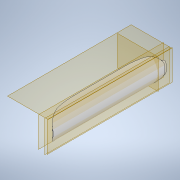
# Autodesk Inventor part: Deckel_Parachute_3
Saved by Autodesk Inventor 2020 (Build 240168000, 168)
## iProperties
Created: 2022-01-25
Part Number: Deckel_Parachute_3
Material: Generisch
Document SubType Name: Modeling
Designer: sp
Density: 1 g/cm^3
Appearance: Vorgabe
Author: sp
## iProperties of the stored document _3D-Druck.ipt
Created: 2022-05-02
Part Number: _3D-Druck
Material: Generisch
Document SubType Name: Modeling
Designer: sp
Density: 1 g/cm^3
Appearance: Vorgabe
Author: sp
Autodesk Inventor part; units mm, degrees
sketch "Skizze1" plane through (0, 0, 0) normal (0, 0, 1) x (1, 0, 0)
  circle A0 centre (0, 0) radius 31
  circle A1 centre (0, 0) radius 30
  dimension "d0" = 62
  dimension "d1" = 60
  constraints: 2 centre point, 2 coincident
  measures "d0" diameter of A0
  measures "d1" diameter of A1
extrude "Extrusion1" add sketch "Skizze1" along normal mid plane 300
sketch "Skizze2" plane through (0, 0, 0) normal (0, 1, 0) x (-1, 0, 0)
  line L0 (-11, 169.5773) -> (-11, -169.8146) construction
  line L1 (-74.8376, 0) -> (82.6362, 0) construction
  line L2 (-11, 75) -> (-11, -75)
  line L3 (-31, -150) -> (-31, 150) projected
  line L4 (31, 150) -> (-31, 150) projected
  line L5 (-31, -150) -> (31, -150) projected
  spline S0 degree 2 poles (-11, 75) (-17.8298, 136.4739) (-72.8449, 128.3193) knots 0 0 0 1 1 1
  spline S1 degree 2 poles (-11, -75) (-17.6171, -136.2673) (-74.8376, -130) knots 0 0 0 1 1 1
  line L6 (-72.8449, 128.3193) -> (-74.8376, -130)
  line L7 (-31, 120) -> (-31, 150)
  line L8 (-31, 150) -> (31, 150)
  line L9 (31, 150) -> (31, -150)
  line L10 (31, -150) -> (31, 150) projected
  line L11 (31, -150) -> (-31, -150)
  line L12 (-31, -150) -> (-31, -120)
  point P0 (0, 0)
  dimension "d4" = 11
  dimension "d5" = 150
  dimension "d6" = 30
  dimension "d7" = 30
  constraints: 18 end point, 5 point on line, 3 perpendicular, 2 collinear, 1 horizontal, 1 symmetric about line, 1 vertical, 6 other
  measures "d4" distance from line of point (0, 0) L0
  measures "d5" distance of L2.start L2.end
  measures "d6" distance from line of L7.start L4
  measures "d7" distance from line of L12.end L5
extrude "Extrusion3" cut sketch "Skizze2" along normal mid plane 100 contours S0 L3 L4 L9 L5 S1 L2
ref_plane "Arbeitsebene1" through (26.5, 0, 0) normal (1, 0, 0) x (0, 1, 0)
sketch "Skizze6" plane through (26.5, 0, 0) normal (1, 0, 0) x (0, 1, 0)
  line L0 (22.6784, 127.732) -> (-25.9609, 127.732)
  line L1 (-25.9609, 127.732) -> (-25.9609, 118.4744)
  line L2 (-25.9609, 118.4744) -> (22.6784, 118.4744)
  line L3 (22.6784, 118.4744) -> (22.6784, 127.732)
  point P0 (0, 0)
  dimension "d27" = 118.4744
  constraints: 8 end point, 2 parallel, 1 horizontal, 1 perpendicular
  measures "d27" distance from line of point (0, 0) L2
extrude "Extrusion5" cut sketch "Skizze6" against normal mid plane 10
ref_plane "Arbeitsebene3" through (0, 33.25, 0) normal (0, 1, 0) x (-1, 0, 0)
mirror "Spiegeln1" about plane through (0, 0, 0) normal (0, 0, 1) of "Extrusion5"
sketch "Skizze8" plane through (0, 33.25, 0) normal (0, 1, 0) x (-1, 0, 0)
  line L0 (-11, -75) -> (-11, 75) projected
  arc A0 (-11, 56.4646) -> (-14.2842, 92.4804) centre (-300.1138, 48.2584) ccw
  arc A1 (-11, 56.4646) -> (-14.2842, 92.4804) centre (-31.6354, 72.7405) ccw
  point P0 (0, 0)
  constraints: 4 point on circle, 2 centre point, 1 point on line
extrude "Extrusion6" cut sketch "Skizze8" against normal blind 65
mirror "Spiegeln2" about plane through (0, 0, 0) normal (0, 0, 1) of "Extrusion6"
ref_plane "Arbeitsebene4" through (0, 0, -103) normal (0, 0, 1) x (1, 0, 0)
sketch "Skizze9" plane through (0, 0, -103) normal (0, 0, 1) x (1, 0, 0)
  circle A0 centre (0, 0) radius 28
  circle A1 centre (0, 0) radius 30
  line L0 (0, 0) -> (55.2327, 31.8886)
  line L1 (0, 0) -> (53.5398, -30.9112)
  line L2 (0, -70.3595) -> (0, 85.9396) construction
  point P0 (24.2487, -14)
  point P1 (25.9808, -15)
  point P2 (25.9808, 15)
  point P3 (24.2487, 14)
  dimension "d36" = 56
  dimension "d37" = 60
  dimension "d38" = 60
  dimension "d39" = 60
  constraints: 6 end point, 2 centre point, 2 coincident, 1 point on line, 1 vertical
  measures "d36" diameter of A0
  measures "d37" diameter of A1
  measures "d38" angle of L0 L1
  measures "d39" angle of L0 L2
extrude "Extrusion7" add sketch "Skizze9" against normal blind 20 contours A0 L0 A1 L1 picked at (29.0396, 3.3572)
fillet "Rundung2" radius 5 2 edges at (25.1147, -14.5, -123) (25.1147, 14.5, -123)
ref_plane "Arbeitsebene5" through (30, 0, 0) normal (1, 0, 0) x (0, 1, 0)
sketch "Skizze10" plane through (30, 0, 0) normal (1, 0, 0) x (0, 1, 0)
  line L0 (0, 194.4728) -> (0, -210.0754) construction
  line L1 (-91.4107, 0) -> (91.4107, 0) construction
  line L2 (-4, 110) -> (4, 110)
  line L3 (4, 110) -> (4, 100)
  line L4 (4, 100) -> (-4, 100)
  line L5 (-4, 100) -> (-4, 110)
  point P0 (0, 0)
  point P1 (0, 0)
  dimension "d44" = 8
  dimension "d45" = 100
  dimension "d46" = 10
  constraints: 12 end point, 2 horizontal, 2 midpoint, 2 parallel, 2 point on line, 1 perpendicular, 1 vertical, 1 other
  measures "d44" distance of L3.end L4.end
  measures "d45" distance between parallel lines of L1 L4
  measures "d46" distance of L2.end L3.end
extrude "Extrusion8" add sketch "Skizze10" against normal blind 11
sketch "Skizze11" plane through (-30, -4, 100) normal (0, -1, 0) x (1, 0, 0)
  line L0 (51, 8) -> (57, 8)
  line L1 (57, 8) -> (57, 2)
  line L2 (57, 2) -> (51, 2)
  line L3 (51, 2) -> (51, 8)
  line L4 (59.7321, 10) -> (49, 10) projected
  line L5 (49, 0) -> (49, 10) projected
  point P0 (30, -100)
  point P1 (0, 10)
  dimension "d49" = 2
  dimension "d50" = 6
  dimension "d51" = 6
  dimension "d52" = 2
  constraints: 8 end point, 2 parallel, 1 horizontal, 1 perpendicular
  measures "d49" distance between parallel lines of L4 L0
  measures "d50" distance of L2.end L0.start
  measures "d51" distance of L0.start L0.end
  measures "d52" distance between parallel lines of L3 L5
extrude "Extrusion9" cut sketch "Skizze11" against normal blind 12
ref_plane "Arbeitsebene6" through (11.5, 0, 0) normal (1, 0, 0) x (0, 1, 0)
sketch "Skizze12" plane through (11.5, 0, 0) normal (1, 0, 0) x (0, 1, 0)
  line L0 (0, 136.0577) -> (0, -137.2687) construction
  line L1 (-53.2386, 0) -> (52.6585, 0) construction
  line L2 (-22.5, 75) -> (-27.5, 75)
  line L3 (-27.5, 75) -> (-27.5, -75)
  line L4 (-27.5, -75) -> (-22.5, -75)
  line L5 (-22.5, -75) -> (-22.5, 75)
  line L6 (22.5, 75) -> (27.5, 75)
  line L7 (27.5, 75) -> (27.5, -75)
  line L8 (27.5, -75) -> (22.5, -75)
  line L9 (22.5, -75) -> (22.5, 75)
  point P0 (0, 0)
  dimension "d56" = 150
  dimension "d57" = 150
  dimension "d58" = 5
  dimension "d59" = 5
  dimension "d60" = 55
  constraints: 20 end point, 4 parallel, 3 horizontal, 2 perpendicular, 2 point on line, 1 vertical, 3 other
  measures "d56" distance of L4.end L2.start
  measures "d57" distance of L6.end L7.end
  measures "d58" distance of L7.end L8.end
  measures "d59" distance of L3.end L4.end
  measures "d60" distance between parallel lines of L7 L3
extrude "Extrusion10" add sketch "Skizze12" along normal blind 2
fillet "Rundung3" radius 2 4 edges at (30, 0, 110) (30, 0, 100) (29.7321, -4, 105) (29.7321, 4, 105)
fillet "Rundung4" radius 2 2 edges at (19, 0, 100) (19, 0, 110)
